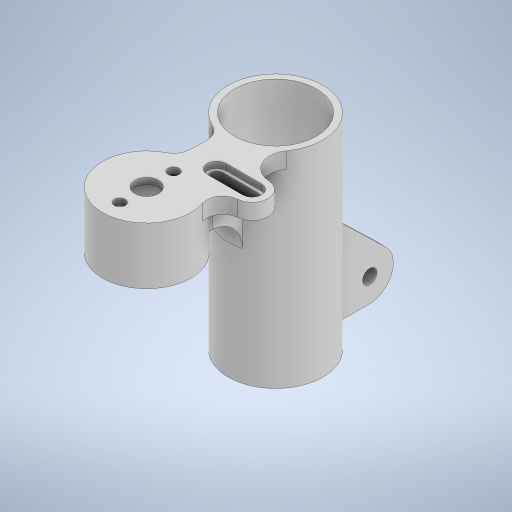
# Autodesk Inventor part: encoderMotorActuatorMount
Saved by Autodesk Inventor 2024.2 (Build 282272000, 272)
## iProperties
Created: 2024-06-06
Part Number: encoderMotorActuatorMount
Material: Generic
Document SubType Name: Modeling
Designer: Robin
Density: 1 g/cm^3
Appearance: Default
Author: Robin
Autodesk Inventor part; units mm, degrees
ref_plane "YZ Plane" through (0, 0, 0) normal (1, 0, 0) x (0, 1, 0)
ref_plane "XZ Plane" through (0, 0, 0) normal (0, 1, 0) x (-1, 0, 0)
ref_plane "XY Plane" through (0, 0, 0) normal (0, 0, 1) x (1, 0, 0)
sketch "Sketch1" plane through (0, 0, 0) normal (0, 1, 0) x (-1, 0, 0)
  circle A0 centre (0, 0) radius 12.75
  circle A1 centre (0, 0) radius 14
  line L0 (4, -12.75) -> (-4, -12.75)
  line L1 (-4, -12.75) -> (-4, -27.75)
  line L2 (-4, -27.75) -> (4, -27.75)
  line L3 (4, -27.75) -> (4, -12.75)
  arc A2 (4, -13.4164) -> (4, -27.75) centre (38.2584, -20.5832) ccw
  point P0 (0, -27.75)
  point P1 (-4, -13.4164)
  point P2 (0, -12.75)
  dimension "d0" = 25.5
  dimension "d1" = 28
  dimension "d2" = 8
  dimension "d3" = 35
  dimension "d5" = 15
  constraints: 8 end point, 4 point on circle, 3 centre point, 2 coincident, 2 parallel, 2 point on line, 1 horizontal, 1 midpoint, 1 perpendicular, 1 tangent, 1 vertical alignment
  measures "d0" diameter of A0
  measures "d1" diameter of A1
  measures "d2" distance of L1.end L2.end
  measures "d3" radius of A2
  measures "d5" distance of L0.end L1.end
extrude "Extrusion1" add sketch "Sketch1" along normal blind 18 contours L0 L1 A1 L3 | L0 L3 A1 L1 | A2 L2 L1 A1
sketch "Sketch2" plane through (0, 18, 0) normal (0, 1, 0) x (1, 0, 0)
  arc A0 (-4, 13.4164) -> (4, 13.4164) centre (0, 0) ccw projected
  circle A1 centre (0, 0) radius 14
  circle A2 centre (0, 0) radius 3.75
  circle A3 centre (0, 8.5) radius 1.75
  circle A4 centre (0, -8.5) radius 1.75
  dimension "d10" = 7.5
  dimension "d11" = 3.5
  dimension "d12" = 3.5
  dimension "d13" = 8.5
  dimension "d14" = 8.5
  constraints: 3 centre point, 2 coincident, 2 vertical alignment, 3 other
  measures "d10" diameter of A2
  measures "d11" diameter of A3
  measures "d12" diameter of A4
  measures "d13" distance of point (0, 0) A3.centre
  measures "d14" distance of point (0, 0) A4.centre
extrude "Extrusion2" add sketch "Sketch2" against normal blind 2
sketch "Sketch3" plane through (0, 0, 0) normal (0, -1, 0) x (1, 0, 0)
  circle A0 centre (0, -40.75) radius 13
  circle A1 centre (0, -40.75) radius 15
  line L0 (4, -27.75) -> (-4, -27.75) projected
  point P0 (0, 0)
  dimension "d15" = 26
  dimension "d16" = 30
  constraints: 2 centre point, 1 coincident, 1 tangent, 1 vertical alignment
  measures "d15" diameter of A0
  measures "d16" diameter of A1
extrude "Extrusion3" add sketch "Sketch3" along normal blind 47 and the other way blind 18
fillet "Fillet1" radius 10 1 edges at (0.1475, 0, -25.7507)
fillet "Fillet2" radius 5 4 edges at (4, 9, -13.4164) (-3.7148, 9, -26.2173) (-3.7148, -5, -26.2173) (-4, 9, -13.4164)
sketch "Sketch5" plane through (0, 18, 0) normal (0, 1, 0) x (1, 0, 0)
  line L0 (4, 16.7332) -> (4, 26.2932) projected
  arc A0 (4, 26.2932) -> (-6.2429, 27.1109) centre (0, 40.75) ccw projected
  arc A1 (-6.2428, 12.5311) -> (6.6316, 12.3297) centre (0, 0) ccw projected
  line L1 (4, 19.5132) -> (4, 23.5132)
  circle A2 centre (0, 0) radius 14
  line L2 (2.3883, 26.9552) -> (2.3883, 13.7948)
  circle A3 centre (0, 40.75) radius 14
  circle A4 centre (0, 40.75) radius 13 projected
  line L3 (2.3883, 14) -> (17.3883, 14)
  line L4 (17.3883, 14) -> (17.3883, 18)
  line L5 (17.3883, 18) -> (2.3883, 18)
  line L6 (2.3883, 18) -> (2.3883, 14)
  circle A5 centre (17.3883, 16) radius 2
  circle A6 centre (17.3883, 16) radius 5
  arc A7 (17.7047, 11.01) -> (13.2787, 4.4358) centre (18.0211, 6.02) ccw
  circle A8 centre (0, 40.75) radius 15 projected
  arc A9 (12.2184, 32.0488) -> (17.61, 20.9951) centre (17.9203, 27.9882) ccw
  point P0 (4, 21.5132)
  point P1 (4, 21.5132)
  point P2 (4, 21.5132)
  point P3 (4, 21.5132)
  point P4 (4, 27.0836)
  point P5 (6.6316, 12.3297)
  point P6 (-6.2428, 12.5311)
  point P7 (-6.1867, 27.9411)
  point P8 (4, 18)
  dimension "d30" = 28
  dimension "d28" = 4
  dimension "d29" = 0
  dimension "d31" = 13.1605
  dimension "d35" = 15
  dimension "d36" = 4
  dimension "d37" = 10
  dimension "d38" = 5
  dimension "d39" = 7
  constraints: 12 end point, 8 point on circle, 5 midpoint, 5 tangent, 4 centre point, 4 coincident, 2 parallel, 1 concentric, 1 horizontal, 1 perpendicular, 1 point on line, 1 vertical, 9 other
  measures "d28" distance of L1.start L1.end
  measures "d29" distance between parallel lines of L0 L1
  measures "d31" distance of L2.start L2.end
  measures "d35" distance of L5.end L4.end
  measures "d36" distance of L3.end L4.end
  measures "d37" diameter of A6
  measures "d38" radius of A7
  measures "d39" radius of A9
extrude "Extrusion4" add sketch "Sketch5" against normal blind 5 contours L0 A0 A9 A6 L5 | A6 L3 A5 L5 | A6 A7 A1 A2 L2 L3 picked at (14.5401, 13.65)
fillet "Fillet4" radius 2 2 edges at (4, 15.5, -18) (4.8132, 15.5, -14)
sketch "Sketch6" plane through (0, 18, 0) normal (0, 1, 0) x (1, 0, 0)
  line L0 (17.3883, 19) -> (6.091, 19)
  line L1 (6.091, 19) -> (6.091, 13)
  line L2 (6.091, 13) -> (17.3883, 13)
  line L3 (17.3883, 13) -> (17.3883, 19)
  circle A0 centre (17.3883, 16) radius 3
  circle A1 centre (6.091, 16) radius 3
  arc A2 (17.3883, 14) -> (17.3883, 18) centre (17.3883, 16) ccw projected
  arc A3 (6.091, 18) -> (6.091, 14) centre (6.091, 16) ccw projected
  point P0 (0, 0)
  point P1 (17.3883, 19)
  point P2 (6.091, 14)
  point P3 (6.091, 18)
  dimension "d41" = 6
  constraints: 8 end point, 2 midpoint, 2 parallel, 1 horizontal, 1 perpendicular, 8 other
  measures "d41" distance between parallel lines of L0 L2
extrude "Extrusion5" cut sketch "Sketch6" against normal blind 2 contours A0 L2 A1 L0 | A0 L3 A2 | L3 A0 | A1 L1 | L1 A3 A1
sketch "Sketch7" plane through (0, -47, -40.75) normal (0, -1, 0) x (1, 0, 0)
  line L0 (2.275, -35) -> (-2.275, -35)
  line L1 (-2.275, -35) -> (-2.275, -13)
  line L2 (-2.275, -13) -> (2.275, -13)
  line L3 (2.275, -13) -> (2.275, -35)
  circle A0 centre (0, 0) radius 13 projected
  point P0 (0, 40.75)
  point P1 (0, -35)
  dimension "d44" = 22
  dimension "d45" = 4.55
  constraints: 8 end point, 2 parallel, 1 horizontal, 1 midpoint, 1 perpendicular, 1 tangent, 1 vertical alignment
  measures "d44" distance of L0.end L1.end
  measures "d45" distance of L0.start L0.end
extrude "Extrusion6" add sketch "Sketch7" against normal blind 30 contours L0 L1 L2 L3
sketch "Sketch8" plane through (-2.275, -47, -75.75) normal (-1, 0, 0) x (0, 0, 1)
  circle A0 centre (7.5, 7.5) radius 7.5
  line L0 (0, 15) -> (15, 15)
  line L1 (15, 15) -> (15, 0)
  line L2 (15, 0) -> (0, 0)
  line L3 (0, 0) -> (0, 15)
  line L4 (20.1735, 0) -> (0, 0) projected
  line L5 (20.1735, 30) -> (20, 30) projected
  line L6 (20, 30) -> (2.2896, 12.8946)
  line L7 (0, 30) -> (20.1735, 30)
  line L8 (20.1735, 30) -> (20.1735, 0)
  line L9 (20.1735, 0) -> (0, 0)
  line L10 (0, 0) -> (0, 30)
  circle A1 centre (7.5, 7.5) radius 2.25
  point P0 (75.75, 47)
  point P1 (0, 7.5)
  point P2 (7.5, 0)
  dimension "d48" = 15
  dimension "d49" = 4.5
  constraints: 18 end point, 5 horizontal, 4 parallel, 2 perpendicular, 2 vertical, 1 centre point, 1 coincident, 1 vertical alignment, 4 other
  measures "d49" diameter of A1
extrude "Extrusion7" cut sketch "Sketch8" against normal blind 30 contours L2 L3 A0 | A0 L3 L0 L6 | L0 L10 L7 L6 | A1
body "Solid1"
